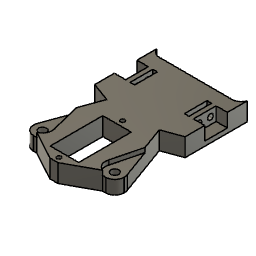
основание (Autodesk Fusion 360 design; units mm, degrees)
Autodesk Fusion 360 part; units mm, degrees
sketch "Sketch1" plane through (0, 0, 0) normal (0, 1, 0) x (1, 0, 0)
  line L0 (-20, 28) -> (20, 28)
  line L1 (20, 28) -> (20, -28)
  line L2 (20, -28) -> (-20, -28)
  line L3 (-20, -28) -> (-20, 28)
  line L4 (-20, 28) -> (20, -28) construction
  line L5 (20, 28) -> (-20, -28) construction
  dimension "d1" = 40
  dimension "d2" = 56
  constraint horizontal L0
  constraint perpendicular L0 L1
  constraint parallel L0 L2
  constraint parallel L1 L3
  constraint coincident L4 origin
  constraint coincident L5 origin
  measures "d1" distance of L1.end L2.end
  measures "d2" distance of L0.end L1.end
extrude "Extrude1" add sketch "Sketch1" along normal blind 8 makes body 1
sketch "Sketch2" plane through (0, 0, -28) normal (0, 0, -1) x (-1, 0, 0)
  line L0 (-20, 0) -> (20, 0)
  line L1 (20, 0) -> (20, 8)
  line L2 (20, 8) -> (-20, 8)
  line L3 (-20, 8) -> (-20, 0)
  line L4 (0, 0) -> (0, 8)
  circle A0 centre (0, 4) radius 2.5
  line L5 (0, 4) -> (-8, 4)
  circle A1 centre (-8, 4) radius 2.5
  line L6 (0, 4) -> (8, 4)
  circle A2 centre (8, 4) radius 2.5
  dimension "d5" = 5
  dimension "d6" = 8
  dimension "d7" = 5
  dimension "d8" = 8
  dimension "d9" = 5
  constraint coincident L4.start origin
  constraint midpoint L2 L4.end
  constraint midpoint L4 A0.centre
  constraint coincident A0.centre L5.start
  constraint perpendicular L4 L5
  constraint coincident L5.end A1.centre
  constraint perpendicular L4 L6
  constraint coincident L6.end A2.centre
  measures "d5" diameter of A0
  measures "d6" distance of A0.centre L5.end
  measures "d7" diameter of A1
  measures "d8" distance of A0.centre L6.end
  measures "d9" diameter of A2
extrude "Extrude2" cut sketch "Sketch2" against normal blind 7 contours L4 A0 L5 | L4 A0 L6 | L4 A0 L5 | L4 A0 L6 | A1 | A2 bodies 1
sketch "Sketch3" plane through (0, 0, -28) normal (0, 0, -1) x (-1, 0, 0)
  circle A0 centre (-8, 4) radius 2.5
  circle A1 centre (0, 4) radius 2.5
  circle A2 centre (8, 4) radius 2.5
  line L0 (-20, 0) -> (20, 0)
  line L1 (20, 0) -> (20, 8)
  line L2 (20, 8) -> (-20, 8)
  line L3 (-20, 8) -> (-20, 0)
  circle A3 centre (-8, 4) radius 3
  circle A4 centre (0, 4) radius 3
  circle A5 centre (8, 4) radius 3
  dimension "d12" = 6
  dimension "d13" = 6
  dimension "d14" = 6
  constraint concentric A0 A3
  constraint concentric A1 A4
  constraint concentric A2 A5
  measures "d12" diameter of A3
  measures "d13" diameter of A4
  measures "d14" diameter of A5
extrude "Extrude3" cut sketch "Sketch3" against normal blind 1 contours A3 | A4 | A5 bodies 1
sketch "Sketch5" plane through (0, 8, 0) normal (0, 1, 0) x (-1, 0, 0)
  line L0 (20, 28) -> (-20, 28)
  line L1 (-20, 28) -> (-20, -28)
  line L2 (-20, -28) -> (20, -28)
  line L3 (20, -28) -> (20, 28)
  line L4 (-20, 28) -> (-20, 18)
  line L5 (-20, 23) -> (-20, 1.5)
  line L6 (-20, 23) -> (-12.6466, 2.7966)
  line L7 (-20, 23) -> (1.5, 23) construction
  line L8 (-20, 28) -> (20, 28)
  line L9 (20, 28) -> (20, 18)
  line L10 (20, 18) -> (-20, 18)
  line L11 (-20, 18) -> (-20, 28)
  line L12 (20, 23) -> (12.6466, 2.7966)
  line L13 (20, 23) -> (-1.5, 23) construction
  line L14 (-12.6466, 2.7966) -> (-11.6205, -0.0225)
  line L15 (12.6466, 2.7966) -> (11.6205, -0.0225)
  line L16 (11.6205, -0.0225) -> (20, -3.0724)
  line L17 (-11.6205, -0.0225) -> (-20, -3.0724)
  dimension "d26" = 10
  dimension "d27" = 21.5
  dimension "d28" = 70
  dimension "d29" = 21.5
  dimension "d30" = 70
  dimension "d31" = 21.5
  dimension "d32" = 3
  dimension "d33" = 3
  constraint coincident L0.end L1.start
  constraint perpendicular L0 L4
  constraint midpoint L4 L5.start
  constraint horizontal L7
  constraint horizontal L8
  constraint vertical L9
  constraint horizontal L10
  constraint vertical L11
  constraint coincident L3 L9.end
  constraint horizontal L13
  constraint midpoint L9 L12.start
  constraint parallel L6 L14
  constraint parallel L12 L15
  constraint coincident L3 L16.end
  constraint perpendicular L15 L16
  constraint coincident L1 L17.end
  constraint perpendicular L14 L17
  measures "d26" distance of L0.end L4.end
  measures "d27" distance of L5.start L5.end
  measures "d28" angle of L6 L7
  measures "d29" distance of L5.start L6.end
  measures "d30" angle of L12 L13
  measures "d31" distance of L12.start L12.end
  measures "d32" distance of L6.end L14.end
  measures "d33" distance of L12.end L15.end
extrude "Extrude5" cut sketch "Sketch5" against normal blind 90 contours L3 L9 L10 L12 | L1 L4 L5 L6 L10 L11 | L3 L10 L12 L15 L16 | L1 L5 L6 L10 L14 L17 bodies 1
sketch "Sketch6" plane through (0, 8, 0) normal (0, 1, 0) x (-1, 0, 0)
  line L0 (-11.6205, -0.0225) -> (-20, -3.0724)
  line L1 (-20, -3.0724) -> (-20, -28)
  line L2 (-20, -28) -> (20, -28)
  line L3 (20, -28) -> (20, -3.0724)
  line L4 (20, -3.0724) -> (11.6205, -0.0225)
  line L5 (11.6205, -0.0225) -> (20, 23)
  line L6 (20, 23) -> (20, 28)
  line L7 (20, 28) -> (-20, 28)
  line L8 (-20, 28) -> (-20, 23)
  line L9 (-20, 23) -> (-11.6205, -0.0225)
  line L10 (-20, 28) -> (-15.9999, 23.9999)
  line L11 (-20, 28) -> (-14.343, 28) construction
  line L12 (20, 28) -> (15.9999, 23.9999)
  line L13 (20, 28) -> (14.343, 28) construction
  circle A0 centre (15.9999, 23.9999) radius 3.15
  circle A1 centre (-15.9999, 23.9999) radius 3.15
  circle A2 centre (15.9999, 23.9999) radius 1.75
  circle A3 centre (-15.9999, 23.9999) radius 1.75
  circle A4 centre (-15.9999, 23.9999) radius 4.0001
  line L14 (-15.9999, 23.9999) -> (-15.9999, 19.9998)
  line L15 (-18.5678, 19.0651) -> (-14.8617, 20.1651)
  circle A5 centre (15.9999, 23.9999) radius 4.0001
  line L16 (15.9999, 23.9999) -> (15.9999, 19.9998)
  line L17 (18.5678, 19.0651) -> (14.8617, 20.1651)
  dimension "d36" = 45
  dimension "d37" = 5.657
  dimension "d38" = 45
  dimension "d39" = 5.657
  dimension "d40" = 6.3
  dimension "d41" = 6.3
  dimension "d42" = 3.5
  dimension "d43" = 3.5
  constraint horizontal L11
  constraint coincident L7.end L8.start
  constraint horizontal L13
  constraint coincident L6.end L7.start
  constraint coincident L12.end A0.centre
  constraint coincident L10.end A1.centre
  constraint concentric A1 A3
  constraint concentric A3 A4
  constraint tangent L7 A4
  constraint coincident A4 L14.end
  constraint vertical L14
  constraint coincident L9 L15.start
  constraint coincident A4 L15.end
  constraint tangent A4 L15
  constraint concentric A0 A5
  constraint tangent L13 A5
  constraint coincident A5 L16.end
  constraint vertical L16
  constraint coincident L5 L17.start
  constraint coincident A5 L17.end
  constraint tangent A5 L17
  measures "d36" angle of L10 L11
  measures "d37" distance of L7.end L10.end
  measures "d38" angle of L12 L13
  measures "d39" distance of L6.end L12.end
  measures "d40" diameter of A0
  measures "d41" diameter of A1
  measures "d42" diameter of A2
  measures "d43" diameter of A3
extrude "Extrude6" cut sketch "Sketch6" against normal blind 6 contours L8 L9 A4 L15 | L10 A1 A4 L14 | L8 L10 A4 | L10 A1 A4 L14 | L7 L10 A4 | L10 A1 A3 L14 | L10 A1 A3 L14 | L10 A3 L14 | L10 A3 L14 | L7 L12 A5 | L12 A0 A5 L16 | L5 L6 A5 L17 | L6 L12 A5 | L12 A0 A5 L16 | L12 A0 A2 L16 | L12 A0 A2 L16 | L12 A2 L16 | L12 A2 L16 bodies 1
extrude "Extrude7" add 2 faces at (-16.9539, 2, 23.7217) (16.9539, 2, 23.7217) along direction (0, -1, 0) blind 4 on bodies 1 bodies 1
extrude "Extrude8" cut 2 faces at (-16.9539, 2, 23.7217) (16.9539, 2, 23.7217) along direction (0, -1, 0) blind 2 on bodies 1 bodies 1
sketch "Sketch7" plane through (0, 0, 0) normal (0, -1, 0) x (1, 0, 0)
  line L0 (18.5678, 19.0651) -> (14.8617, 20.1651)
  arc A0 (15.9999, 28) -> (14.8617, 20.1651) centre (15.9999, 23.9999) ccw
  line L1 (15.9999, 28) -> (-15.9999, 28)
  arc A1 (-14.8617, 20.1651) -> (-15.9999, 28) centre (-15.9999, 23.9999) ccw
  line L2 (-14.8617, 20.1651) -> (-18.5678, 19.0651)
  line L3 (-18.5678, 19.0651) -> (-11.6205, -0.0225)
  line L4 (-11.6205, -0.0225) -> (-20, -3.0724)
  line L5 (-20, -3.0724) -> (-20, -28)
  line L6 (-20, -28) -> (20, -28)
  line L7 (20, -28) -> (20, -3.0724)
  line L8 (20, -3.0724) -> (11.6205, -0.0225)
  line L9 (11.6205, -0.0225) -> (18.5678, 19.0651)
  circle A2 centre (-15.9999, 23.9999) radius 5.5629
  circle A3 centre (15.9999, 23.9999) radius 5.5629
  constraint concentric A1 A2
  constraint coincident L2.end A2
  constraint concentric A0 A3
  constraint coincident L0.start A3
sketch "Sketch10" plane through (0, 8, 0) normal (0, 1, 0) x (-1, 0, 0)
  arc A0 (15.9999, 28) -> (14.8617, 20.1651) centre (15.9999, 23.9999) ccw
  line L0 (15.9999, 28) -> (-15.9999, 28)
  arc A1 (-14.8617, 20.1651) -> (-15.9999, 28) centre (-15.9999, 23.9999) ccw
  line L1 (-14.8617, 20.1651) -> (-18.5678, 19.0651)
  line L2 (-18.5678, 19.0651) -> (-11.6205, -0.0225)
  line L3 (-11.6205, -0.0225) -> (-20, -3.0724)
  line L4 (-20, -3.0724) -> (-20, -28)
  line L5 (-20, -28) -> (20, -28)
  line L6 (20, -28) -> (20, -3.0724)
  line L7 (20, -3.0724) -> (11.6205, -0.0225)
  line L8 (11.6205, -0.0225) -> (18.5678, 19.0651)
  line L9 (18.5678, 19.0651) -> (14.8617, 20.1651)
  line L10 (-20, -28) -> (20, -28)
  line L11 (20, -28) -> (20, -55)
  line L12 (20, -55) -> (-20, -55)
  line L13 (-20, -55) -> (-20, -28)
  constraint horizontal L10
  constraint vertical L11
  constraint horizontal L12
  constraint vertical L13
  constraint coincident L4.end L5.start
extrude "Extrude12" add sketch "Sketch10" against normal blind 7 separate body contours L5 L10 L11 L12 L13 makes body 2
sketch "Sketch11" plane through (0, 8, 0) normal (0, 1, 0) x (-1, 0, 0)
  line L0 (-20, -55) -> (20, -55)
  line L1 (20, -55) -> (20, -28)
  line L2 (20, -28) -> (-20, -28)
  line L3 (-20, -28) -> (-20, -55)
  line L4 (20, -28) -> (15.9999, -32.0001)
  line L5 (20, -28) -> (14.343, -28) construction
  line L6 (-20, -28) -> (-15.9999, -32.0001)
  line L7 (-20, -28) -> (-14.343, -28) construction
  circle A0 centre (15.9999, -32.0001) radius 4.0001
  circle A1 centre (-15.9999, -32.0001) radius 4.0001
  dimension "d63" = 45
  dimension "d64" = 5.657
  dimension "d65" = 5.657
  dimension "d66" = 45
  constraint horizontal L5
  constraint coincident L1.end L2.start
  constraint horizontal L7
  constraint coincident L2.end L3.start
  constraint coincident L4.end A0.centre
  constraint tangent L5 A0
  constraint coincident L6.end A1.centre
  constraint tangent L7 A1
  measures "d63" angle of L4 L5
  measures "d64" distance of L1.end L4.end
  measures "d65" distance of L2.end L6.end
  measures "d66" angle of L6 L7
extrude "Extrude13" cut sketch "Sketch11" against normal blind 25 contours L0 L1 L2 L3 A0 A1 | A1 | A0 bodies 2 makes body 3 at (19.4641, 3.3333, -30.0001)
extrude "Extrude14" add 2 faces at (19.2141, 1, -28.7859) (-19.2141, 1, -28.7859) along direction (0, -1, 0) blind 1 on bodies 2 3 bodies 3 1 2
sketch "Sketch12" plane through (0, 8, 0) normal (0, 1, 0) x (-1, 0, 0)
  arc A0 (-15.9999, -28) -> (-20, -32.0001) centre (-15.9999, -32.0001) ccw
  line L0 (-15.9999, -28) -> (15.9999, -28)
  arc A1 (20, -32.0001) -> (15.9999, -28) centre (15.9999, -32.0001) ccw
  line L1 (20, -32.0001) -> (20, -3.0724)
  line L2 (20, -3.0724) -> (11.6205, -0.0225)
  line L3 (11.6205, -0.0225) -> (18.5678, 19.0651)
  line L4 (18.5678, 19.0651) -> (14.8617, 20.1651)
  arc A2 (15.9999, 28) -> (14.8617, 20.1651) centre (15.9999, 23.9999) ccw
  line L5 (15.9999, 28) -> (-15.9999, 28)
  arc A3 (-14.8617, 20.1651) -> (-15.9999, 28) centre (-15.9999, 23.9999) ccw
  line L6 (-14.8617, 20.1651) -> (-18.5678, 19.0651)
  line L7 (-18.5678, 19.0651) -> (-11.6205, -0.0225)
  line L8 (-11.6205, -0.0225) -> (-20, -3.0724)
  line L9 (-20, -3.0724) -> (-20, -32.0001)
  circle A4 centre (-15.9999, -32.0001) radius 4.25
  circle A5 centre (15.9999, -32.0001) radius 4.25
  dimension "d71" = 8.5
  dimension "d72" = 8.5
  constraint concentric A0 A4
  constraint concentric A1 A5
  measures "d71" diameter of A4
  measures "d72" diameter of A5
extrude "Extrude15" cut sketch "Sketch12" against normal blind 16 contours A0 L0 L9 A4 | L0 A1 L1 A5 picked at (-16.8835, -28.0205) picked at (19.8255, -30.5919) bodies 3
sketch "Sketch13" plane through (0, 8, 0) normal (0, 1, 0) x (-1, 0, 0)
  arc A0 (-14.564, -28) -> (-20, -30.5642) centre (-15.9999, -32.0001) ccw
  line L0 (-14.564, -28) -> (14.564, -28)
  arc A1 (20, -30.5642) -> (14.564, -28) centre (15.9999, -32.0001) ccw
  line L1 (20, -30.5642) -> (20, -3.0724)
  line L2 (20, -3.0724) -> (11.6205, -0.0225)
  line L3 (11.6205, -0.0225) -> (18.5678, 19.0651)
  line L4 (18.5678, 19.0651) -> (14.8617, 20.1651)
  arc A2 (15.9999, 28) -> (14.8617, 20.1651) centre (15.9999, 23.9999) ccw
  line L5 (15.9999, 28) -> (-15.9999, 28)
  arc A3 (-14.8617, 20.1651) -> (-15.9999, 28) centre (-15.9999, 23.9999) ccw
  line L6 (-14.8617, 20.1651) -> (-18.5678, 19.0651)
  line L7 (-18.5678, 19.0651) -> (-11.6205, -0.0225)
  line L8 (-11.6205, -0.0225) -> (-20, -3.0724)
  line L9 (-20, -3.0724) -> (-20, -30.5642)
  line L10 (0, -28) -> (-20, -28)
  line L11 (-15.99, -28) -> (-15.99, -27.7501)
  line L12 (-15.99, -27.7501) -> (-20, -27.7408)
  line L13 (-15.99, -27.7501) -> (20, -27.8339)
  constraint midpoint L0 L10.start
  constraint coincident L9 L10.end
  constraint perpendicular L9 L10
  constraint coincident L10 L11.start
  constraint coincident A0 L11.end
  constraint perpendicular L10 L11
  constraint coincident L9 L12.end
  constraint tangent A0 L12
  constraint coincident L1 L13.end
  constraint tangent A0 L13
extrude "Extrude16" cut sketch "Sketch13" against normal blind 17 contours A0 L0 A1 L10 L13 bodies 3
extrude "Extrude17" cut 3 faces at (-10.8222, 3.851, -27) (-2.8222, 3.851, -27) (5.1871, 3.7268, -27) along direction (0, 0, 1) blind 0.2 on bodies 3 bodies 3
extrude "Extrude18" add 2 faces at (-16.9539, 0, 23.7217) (16.9539, 0, 23.7217) along direction (0, 1, 0) blind 8 on bodies 3 bodies 3
extrude "Extrude19" cut 2 faces at (-16.9539, -2, 23.7217) (16.9539, -2, 23.7217) along direction (0, 1, 0) blind 2 on bodies 3 bodies 3
sketch "Sketch14" plane through (0, 8, 0) normal (0, 1, 0) x (-1, 0, 0)
  line L0 (-15.99, -27.7501) -> (15.2175, -27.8227)
  arc A0 (20, -30.5642) -> (15.2175, -27.8227) centre (15.9999, -32.0001) ccw
  line L1 (20, -30.5642) -> (20, -3.0724)
  line L2 (20, -3.0724) -> (11.6205, -0.0225)
  line L3 (11.6205, -0.0225) -> (20, 23)
  line L4 (20, 23) -> (20, 28)
  line L5 (20, 28) -> (-20, 28)
  line L6 (-20, 28) -> (-20, 23)
  line L7 (-20, 23) -> (-11.6205, -0.0225)
  line L8 (-11.6205, -0.0225) -> (-20, -3.0724)
  line L9 (-20, -3.0724) -> (-20, -30.5642)
  arc A1 (-15.99, -27.7501) -> (-20, -30.5642) centre (-15.9999, -32.0001) ccw
  line L10 (20, 28) -> (15.9999, 23.9999)
  line L11 (20, 28) -> (14.343, 28) construction
  line L12 (-20, 28) -> (-15.9999, 23.9999)
  line L13 (-20, 28) -> (-14.343, 28) construction
  circle A2 centre (15.9999, 23.9999) radius 1.75
  circle A3 centre (-15.9999, 23.9999) radius 1.75
  circle A4 centre (15.9999, 23.9999) radius 4.0001
  circle A5 centre (-15.9999, 23.9999) radius 4.0001
  dimension "d83" = 45
  dimension "d84" = 5.657
  dimension "d85" = 5.657
  dimension "d86" = 45
  dimension "d87" = 3.5
  dimension "d88" = 3.5
  constraint horizontal L11
  constraint coincident L4.end L5.start
  constraint horizontal L13
  constraint coincident L5.end L6.start
  constraint coincident L10.end A2.centre
  constraint coincident L12.end A3.centre
  constraint concentric A2 A4
  constraint tangent L4 A4
  constraint concentric A3 A5
  constraint tangent L6 A5
  measures "d83" angle of L10 L11
  measures "d84" distance of L4.end L10.end
  measures "d85" distance of L5.end L12.end
  measures "d86" angle of L12 L13
  measures "d87" diameter of A2
  measures "d88" diameter of A3
extrude "Extrude20" cut sketch "Sketch14" against normal blind 90 contours L6 L12 A5 | L4 L10 A4 | L5 L12 A5 | L5 L10 A4 | A2 | A3 bodies 3
fillet "Fillet1" radius 5 2 edges at (-20, 4, 23) (20, 4, 23) on bodies 3
sketch "Sketch15" plane through (0, 8, 0) normal (0, 1, 0) x (-1, 0, 0)
  arc A0 (-20, 23.8816) -> (-19.6985, 22.1715) centre (-15, 23.8816) ccw
  line L0 (-19.6985, 22.1715) -> (-11.6205, -0.0225)
  line L1 (-11.6205, -0.0225) -> (-20, -3.0724)
  line L2 (-20, -3.0724) -> (-20, -30.5642)
  arc A1 (-15.99, -27.7501) -> (-20, -30.5642) centre (-15.9999, -32.0001) ccw
  line L3 (-15.99, -27.7501) -> (15.2175, -27.8227)
  arc A2 (20, -30.5642) -> (15.2175, -27.8227) centre (15.9999, -32.0001) ccw
  line L4 (20, -30.5642) -> (20, -3.0724)
  line L5 (20, -3.0724) -> (11.6205, -0.0225)
  line L6 (11.6205, -0.0225) -> (19.6985, 22.1715)
  arc A3 (19.6985, 22.1715) -> (20, 23.8816) centre (15, 23.8816) ccw
  line L7 (20, 23.8816) -> (20, 23.9999)
  arc A4 (20, 23.9999) -> (15.9999, 28) centre (15.9999, 23.9999) ccw
  line L8 (15.9999, 28) -> (-15.9999, 28)
  arc A5 (-15.9999, 28) -> (-20, 23.9999) centre (-15.9999, 23.9999) ccw
  line L9 (-20, 23.9999) -> (-20, 23.8816)
  circle A6 centre (-15.9999, 23.9999) radius 1.75
  circle A7 centre (15.9999, 23.9999) radius 1.75
  circle A8 centre (15.9999, 23.9999) radius 4.25
  circle A9 centre (-15.9999, 23.9999) radius 4.25
  dimension "d94" = 8.5
  dimension "d95" = 8.5
  constraint concentric A4 A8
  constraint concentric A5 A9
  measures "d94" diameter of A8
  measures "d95" diameter of A9
extrude "Extrude21" cut sketch "Sketch15" against normal blind 2 contours A0 L0 L8 A5 L9 A9 | L6 A3 L7 A4 L8 A8 picked at (-15.3915, 27.2353) picked at (15.3915, 27.2353) bodies 3
sketch "Sketch16" plane through (0, 8, 0) normal (0, 1, 0) x (-1, 0, 0)
  arc A0 (14.564, 28) -> (19.4717, 21.5486) centre (15.9999, 23.9999) ccw
  line L0 (14.564, 28) -> (-14.564, 28)
  arc A1 (-19.4717, 21.5486) -> (-14.564, 28) centre (-15.9999, 23.9999) ccw
  line L1 (-19.4717, 21.5486) -> (-11.6205, -0.0225)
  line L2 (-11.6205, -0.0225) -> (-20, -3.0724)
  line L3 (-20, -3.0724) -> (-20, -30.5642)
  arc A2 (-15.99, -27.7501) -> (-20, -30.5642) centre (-15.9999, -32.0001) ccw
  line L4 (-15.99, -27.7501) -> (15.2175, -27.8227)
  arc A3 (20, -30.5642) -> (15.2175, -27.8227) centre (15.9999, -32.0001) ccw
  line L5 (20, -30.5642) -> (20, -3.0724)
  line L6 (20, -3.0724) -> (11.6205, -0.0225)
  line L7 (11.6205, -0.0225) -> (19.4717, 21.5486)
  line L8 (15.9999, 23.9999) -> (11.7499, 23.9999)
  line L9 (15.9999, 23.9999) -> (15.9999, 19.7499)
  line L10 (15.9999, 19.7499) -> (16.5, 19.7499)
  line L11 (16.5, 19.7499) -> (18.8171, 19.7499)
  constraint coincident A0.centre L8.start
  constraint coincident A0 L8.end
  constraint horizontal L8
  constraint coincident A0 L9.end
  constraint perpendicular L8 L9
  constraint tangent A0 L10
  constraint coincident L7 L11.end
  constraint perpendicular L9 L11
extrude "Extrude22" cut sketch "Sketch16" against normal blind 2 contours A0 L7 L10 L11 bodies 3
sketch "Sketch17" plane through (0, 8, 0) normal (0, 1, 0) x (-1, 0, 0)
  line L0 (18.8171, 19.7499) -> (15.9999, 19.7499)
  arc A0 (14.564, 28) -> (15.9999, 19.7499) centre (15.9999, 23.9999) ccw
  line L1 (14.564, 28) -> (-14.564, 28)
  arc A1 (-19.4717, 21.5486) -> (-14.564, 28) centre (-15.9999, 23.9999) ccw
  line L2 (-19.4717, 21.5486) -> (-11.6205, -0.0225)
  line L3 (-11.6205, -0.0225) -> (-20, -3.0724)
  line L4 (-20, -3.0724) -> (-20, -30.5642)
  arc A2 (-15.99, -27.7501) -> (-20, -30.5642) centre (-15.9999, -32.0001) ccw
  line L5 (-15.99, -27.7501) -> (15.2175, -27.8227)
  arc A3 (20, -30.5642) -> (15.2175, -27.8227) centre (15.9999, -32.0001) ccw
  line L6 (20, -30.5642) -> (20, -3.0724)
  line L7 (20, -3.0724) -> (11.6205, -0.0225)
  line L8 (11.6205, -0.0225) -> (18.8171, 19.7499)
  line L9 (-15.9999, 23.9999) -> (-15.9999, 19.7499)
  line L10 (-15.9999, 19.7499) -> (-18.8171, 19.7499)
  constraint coincident A1.centre L9.start
  constraint coincident A1 L9.end
  constraint coincident L2 L10.end
  constraint tangent A1 L10
extrude "Extrude23" cut sketch "Sketch17" against normal blind 2 contours A1 L2 L10 bodies 3
sketch "Sketch18" plane through (0, 8, 0) normal (0, 1, 0) x (-1, 0, 0)
  line L0 (-15.9999, 19.7499) -> (-18.8171, 19.7499)
  line L1 (-18.8171, 19.7499) -> (-11.6205, -0.0225)
  line L2 (-11.6205, -0.0225) -> (-20, -3.0724)
  line L3 (-20, -3.0724) -> (-20, -30.5642)
  arc A0 (-15.99, -27.7501) -> (-20, -30.5642) centre (-15.9999, -32.0001) ccw
  line L4 (-15.99, -27.7501) -> (15.2175, -27.8227)
  arc A1 (20, -30.5642) -> (15.2175, -27.8227) centre (15.9999, -32.0001) ccw
  line L5 (20, -30.5642) -> (20, -3.0724)
  line L6 (20, -3.0724) -> (11.6205, -0.0225)
  line L7 (11.6205, -0.0225) -> (18.8171, 19.7499)
  line L8 (18.8171, 19.7499) -> (15.9999, 19.7499)
  arc A2 (14.564, 28) -> (15.9999, 19.7499) centre (15.9999, 23.9999) ccw
  line L9 (14.564, 28) -> (-14.564, 28)
  arc A3 (-15.9999, 19.7499) -> (-14.564, 28) centre (-15.9999, 23.9999) ccw
  line L10 (-0.3862, -27.7864) -> (20, -27.7864)
  line L11 (20, -27.7864) -> (20.014, -21.7864)
  line L12 (20.014, -21.7864) -> (15.014, -21.7864)
  line L13 (15.014, -21.7864) -> (15.014, -11.7864)
  line L14 (15.014, -11.7864) -> (20.014, -11.7864)
  line L15 (20.014, -11.7864) -> (20.014, -21.7864)
  line L16 (15.014, -21.7864) -> (-20, -21.7864)
  line L17 (-20, -21.7864) -> (-15, -21.7864)
  line L18 (-15, -21.7864) -> (-15, -11.7864)
  line L19 (-15, -11.7864) -> (-20, -11.7864)
  line L20 (-20, -11.7864) -> (-20, -21.7864)
  dimension "d102" = 6
  dimension "d103" = 5
  dimension "d104" = 10
  dimension "d105" = 5
  dimension "d106" = 10
  constraint midpoint L4 L10.start
  constraint coincident L5 L10.end
  constraint perpendicular L5 L10
  constraint perpendicular L4 L11
  constraint horizontal L12
  constraint vertical L13
  constraint horizontal L14
  constraint vertical L15
  constraint coincident L3 L16.end
  constraint perpendicular L3 L16
  constraint horizontal L17
  constraint vertical L18
  constraint horizontal L19
  constraint vertical L20
  measures "d102" distance of L10.end L11.end
  measures "d103" distance of L11.end L12.end
  measures "d104" distance of L11.end L14.end
  measures "d105" distance of L16.end L17.end
  measures "d106" distance of L16.end L19.end
extrude "Extrude24" cut sketch "Sketch18" against normal blind 6 contours L3 L16 L17 L18 L19 L20 | L5 L12 L13 L14 bodies 3
sketch "Sketch19" plane through (-15.014, 0, 0) normal (-1, 0, 0) x (0, 0, 1)
  line L0 (-11.7864, 8) -> (-21.7864, 8)
  line L1 (-21.7864, 8) -> (-21.7864, 2)
  line L2 (-21.7864, 2) -> (-11.7864, 2)
  line L3 (-11.7864, 2) -> (-11.7864, 8)
  line L4 (-21.7864, 8) -> (-21.7864, 2)
  line L5 (-21.7864, 5) -> (-19.2864, 5)
  line L6 (-11.7864, 5) -> (-14.2864, 5)
  circle A0 centre (-19.2864, 5) radius 1.25
  circle A1 centre (-14.2864, 5) radius 1.25
  dimension "d109" = 2.5
  dimension "d110" = 2.5
  dimension "d111" = 2.5
  dimension "d112" = 2.5
  constraint coincident L0.end L1.start
  constraint coincident L1.end L2.start
  constraint midpoint L4 L5.start
  constraint perpendicular L4 L5
  constraint midpoint L3 L6.start
  constraint perpendicular L3 L6
  constraint coincident L5.end A0.centre
  constraint coincident L6.end A1.centre
  measures "d109" distance of L5.start L5.end
  measures "d110" distance of L6.start L6.end
  measures "d111" diameter of A0
  measures "d112" diameter of A1
extrude "Extrude25" cut sketch "Sketch19" against normal blind 4 contours A0 | A1 bodies 3
sketch "Sketch20" plane through (0, 8, 0) normal (0, 1, 0) x (-1, 0, 0)
  line L0 (-20, -11.7864) -> (-15, -11.7864)
  line L1 (-15, -11.7864) -> (-15, -21.7864)
  line L2 (-15, -21.7864) -> (-20, -21.7864)
  line L3 (-20, -21.7864) -> (-20, -30.5642)
  arc A0 (-15.99, -27.7501) -> (-20, -30.5642) centre (-15.9999, -32.0001) ccw
  line L4 (-15.99, -27.7501) -> (15.2175, -27.8227)
  arc A1 (20, -30.5642) -> (15.2175, -27.8227) centre (15.9999, -32.0001) ccw
  line L5 (20, -30.5642) -> (20, -21.7864)
  line L6 (20, -21.7864) -> (15.014, -21.7864)
  line L7 (15.014, -21.7864) -> (15.014, -11.7864)
  line L8 (15.014, -11.7864) -> (20, -11.7864)
  line L9 (20, -11.7864) -> (20, -3.0724)
  line L10 (20, -3.0724) -> (11.6205, -0.0225)
  line L11 (11.6205, -0.0225) -> (18.8171, 19.7499)
  line L12 (18.8171, 19.7499) -> (15.9999, 19.7499)
  arc A2 (14.564, 28) -> (15.9999, 19.7499) centre (15.9999, 23.9999) ccw
  line L13 (14.564, 28) -> (-14.564, 28)
  arc A3 (-15.9999, 19.7499) -> (-14.564, 28) centre (-15.9999, 23.9999) ccw
  line L14 (-15.9999, 19.7499) -> (-18.8171, 19.7499)
  line L15 (-18.8171, 19.7499) -> (-11.6205, -0.0225)
  line L16 (-11.6205, -0.0225) -> (-20, -3.0724)
  line L17 (-20, -3.0724) -> (-20, -11.7864)
  line L18 (20, -21.7864) -> (15.014, -21.7864)
  line L19 (15.014, -21.7864) -> (11.014, -21.7864)
  line L20 (15.014, -21.7864) -> (15.014, -19.2864)
  line L21 (15.014, -19.2864) -> (11.014, -19.2864)
  line L22 (11.014, -19.2864) -> (13.014, -19.2864)
  line L23 (12.014, -19.2864) -> (12.014, -21.7864)
  line L24 (12.014, -21.7864) -> (12.014, -16.7864)
  line L25 (11.014, -21.7864) -> (13.014, -21.7864)
  line L26 (13.014, -21.7864) -> (13.014, -16.7864)
  line L27 (13.014, -16.7864) -> (11.014, -16.7864)
  line L28 (11.014, -16.7864) -> (11.014, -21.7864)
  line L29 (15.014, -11.7864) -> (15.014, -14.2864)
  line L30 (15.014, -14.2864) -> (12.014, -14.2864)
  line L31 (12.014, -14.2864) -> (12.014, -11.7864)
  line L32 (13.014, -11.7864) -> (11.014, -11.7864)
  line L33 (11.014, -11.7864) -> (11.014, -16.7864)
  line L34 (11.014, -16.7864) -> (13.014, -16.7864)
  line L35 (13.014, -16.7864) -> (13.014, -11.7864)
  line L36 (13.014, -11.7864) -> (11.014, -16.7864) construction
  line L37 (11.014, -11.7864) -> (13.014, -16.7864) construction
  point P0 (12.014, -14.2864)
  dimension "d115" = 4
  dimension "d116" = 2.5
  dimension "d117" = 4
  dimension "d118" = 2
  dimension "d119" = 2.5
  dimension "d120" = 5
  dimension "d121" = 2.5
  dimension "d122" = 2.5
  dimension "d123" = 2
  constraint coincident L5.end L6.start
  constraint coincident L6.end L7.start
  constraint perpendicular L5 L19
  constraint perpendicular L6 L20
  constraint perpendicular L20 L21
  constraint parallel L21 L22
  constraint midpoint L22 L23.start
  constraint perpendicular L21 L23
  constraint perpendicular L19 L24
  constraint horizontal L25
  constraint vertical L26
  constraint horizontal L27
  constraint vertical L28
  constraint coincident L7.end L8.start
  constraint perpendicular L8 L29
  constraint perpendicular L29 L30
  constraint perpendicular L30 L31
  constraint horizontal L32
  constraint perpendicular L32 L33
  constraint parallel L32 L34
  constraint parallel L33 L35
  constraint coincident L36 P0
  constraint coincident L37 P0
  constraint coincident P0 L30.end
  measures "d115" distance of L6.end L19.end
  measures "d116" distance of L6.end L20.end
  measures "d117" distance of L20.end L21.end
  measures "d118" distance of L21.end L22.end
  measures "d119" distance of L23.start L23.end
  measures "d120" distance of L23.end L24.end
  measures "d121" distance of L7.end L29.end
  measures "d122" distance of P0 L31.end
  measures "d123" distance of L27.end L26.end
extrude "Extrude26" cut sketch "Sketch20" against normal blind 5 contours L19 L21 L22 L23 L24 L25 L26 | L21 L22 L24 L26 L27 L34 | L19 L21 L22 L23 L24 L25 L28 | L27 L30 L31 L32 L33 L34 L35 | L30 L31 L32 L35 | L21 L22 L24 L27 L28 L34 bodies 3
sketch "Sketch21" plane through (0, 8, 0) normal (0, 1, 0) x (-1, 0, 0)
  line L0 (11.014, -11.7864) -> (13.014, -11.7864)
  line L1 (13.014, -11.7864) -> (13.014, -21.7864)
  line L2 (13.014, -21.7864) -> (11.014, -21.7864)
  line L3 (11.014, -21.7864) -> (11.014, -11.7864)
  line L4 (-20, -11.7864) -> (-15, -11.7864)
  line L5 (-15, -11.7864) -> (-15, -21.7864)
  line L6 (-15, -21.7864) -> (-20, -21.7864)
  line L7 (-20, -21.7864) -> (-20, -30.5642)
  arc A0 (-15.99, -27.7501) -> (-20, -30.5642) centre (-15.9999, -32.0001) ccw
  line L8 (-15.99, -27.7501) -> (15.2175, -27.8227)
  arc A1 (20, -30.5642) -> (15.2175, -27.8227) centre (15.9999, -32.0001) ccw
  line L9 (20, -30.5642) -> (20, -21.7864)
  line L10 (20, -21.7864) -> (15.014, -21.7864)
  line L11 (15.014, -21.7864) -> (15.014, -11.7864)
  line L12 (15.014, -11.7864) -> (20, -11.7864)
  line L13 (20, -11.7864) -> (20, -3.0724)
  line L14 (20, -3.0724) -> (11.6205, -0.0225)
  line L15 (11.6205, -0.0225) -> (18.8171, 19.7499)
  line L16 (18.8171, 19.7499) -> (15.9999, 19.7499)
  arc A2 (14.564, 28) -> (15.9999, 19.7499) centre (15.9999, 23.9999) ccw
  line L17 (14.564, 28) -> (-14.564, 28)
  arc A3 (-15.9999, 19.7499) -> (-14.564, 28) centre (-15.9999, 23.9999) ccw
  line L18 (-15.9999, 19.7499) -> (-18.8171, 19.7499)
  line L19 (-18.8171, 19.7499) -> (-11.6205, -0.0225)
  line L20 (-11.6205, -0.0225) -> (-20, -3.0724)
  line L21 (-20, -3.0724) -> (-20, -11.7864)
  line L22 (-15, -16.7864) -> (-13, -16.7864)
  line L23 (-13, -16.7864) -> (-13, -11.7864)
  line L24 (-13, -11.7864) -> (-11, -11.7864)
  line L25 (-11, -11.7864) -> (-11, -21.7864)
  line L26 (-11, -21.7864) -> (-13, -21.7864)
  line L27 (-13, -21.7864) -> (-13, -11.7864)
  dimension "d126" = 2
  dimension "d127" = 2
  dimension "d128" = 10
  constraint midpoint L5 L22.start
  constraint perpendicular L5 L22
  constraint perpendicular L22 L23
  constraint horizontal L24
  constraint vertical L25
  constraint horizontal L26
  constraint vertical L27
  measures "d126" distance of L22.start L22.end
  measures "d127" distance of L23.end L24.end
  measures "d128" distance of L23.end L26.end
extrude "Extrude27" cut sketch "Sketch21" against normal blind 5 contours L23 L24 L25 L26 L27 bodies 3
sketch "Sketch22" plane through (15, 0, 0) normal (1, 0, 0) x (0, 0, -1)
  line L0 (21.7864, 8) -> (11.7864, 8)
  line L1 (11.7864, 8) -> (11.7864, 2)
  line L2 (11.7864, 2) -> (21.7864, 2)
  line L3 (21.7864, 2) -> (21.7864, 8)
  line L4 (11.7864, 5) -> (14.2864, 5)
  circle A0 centre (14.2864, 5) radius 1.25
  line L5 (21.7864, 5) -> (19.2864, 5)
  circle A1 centre (19.2864, 5) radius 1.25
  dimension "d131" = 2.5
  dimension "d132" = 2.5
  dimension "d133" = 2.5
  dimension "d134" = 2.5
  constraint midpoint L1 L4.start
  constraint perpendicular L1 L4
  constraint coincident L4.end A0.centre
  constraint midpoint L3 L5.start
  constraint perpendicular L3 L5
  constraint coincident L5.end A1.centre
  measures "d131" distance of L4.start L4.end
  measures "d132" diameter of A0
  measures "d133" distance of L5.start L5.end
  measures "d134" diameter of A1
extrude "Extrude28" cut sketch "Sketch22" against normal blind 4 contours A0 | A1 bodies 3
sketch "Sketch23" plane through (0, 8, 0) normal (0, 1, 0) x (-1, 0, 0)
  line L0 (-11, -11.7864) -> (-11, -21.7864)
  line L1 (-11, -21.7864) -> (-13, -21.7864)
  line L2 (-13, -21.7864) -> (-13, -11.7864)
  line L3 (-13, -11.7864) -> (-11, -11.7864)
  line L4 (11.014, -11.7864) -> (13.014, -11.7864)
  line L5 (13.014, -11.7864) -> (13.014, -21.7864)
  line L6 (13.014, -21.7864) -> (11.014, -21.7864)
  line L7 (11.014, -21.7864) -> (11.014, -11.7864)
  line L8 (-20, -11.7864) -> (-15, -11.7864)
  line L9 (-15, -11.7864) -> (-15, -21.7864)
  line L10 (-15, -21.7864) -> (-20, -21.7864)
  line L11 (-20, -21.7864) -> (-20, -30.5642)
  arc A0 (-15.99, -27.7501) -> (-20, -30.5642) centre (-15.9999, -32.0001) ccw
  line L12 (-15.99, -27.7501) -> (15.2175, -27.8227)
  arc A1 (20, -30.5642) -> (15.2175, -27.8227) centre (15.9999, -32.0001) ccw
  line L13 (20, -30.5642) -> (20, -21.7864)
  line L14 (20, -21.7864) -> (15.014, -21.7864)
  line L15 (15.014, -21.7864) -> (15.014, -11.7864)
  line L16 (15.014, -11.7864) -> (20, -11.7864)
  line L17 (20, -11.7864) -> (20, -3.0724)
  line L18 (20, -3.0724) -> (11.6205, -0.0225)
  line L19 (11.6205, -0.0225) -> (18.8171, 19.7499)
  line L20 (18.8171, 19.7499) -> (15.9999, 19.7499)
  arc A2 (14.564, 28) -> (15.9999, 19.7499) centre (15.9999, 23.9999) ccw
  line L21 (14.564, 28) -> (-14.564, 28)
  arc A3 (-15.9999, 19.7499) -> (-14.564, 28) centre (-15.9999, 23.9999) ccw
  line L22 (-15.9999, 19.7499) -> (-18.8171, 19.7499)
  line L23 (-18.8171, 19.7499) -> (-11.6205, -0.0225)
  line L24 (-11.6205, -0.0225) -> (-20, -3.0724)
  line L25 (-20, -3.0724) -> (-20, -11.7864)
  line L26 (-11.8128, 23.2712) -> (-15.2188, 9.8637)
  line L27 (11.8128, 23.2712) -> (15.2188, 9.8637)
  constraint midpoint A3 L26.start
  constraint midpoint L23 L26.end
  constraint midpoint A2 L27.start
  constraint midpoint L19 L27.end
extrude "Extrude29" cut sketch "Sketch23" against normal blind 2 contours A3 L22 L23 L26 | L19 L20 A2 L27 bodies 3
sketch "Sketch24" plane through (0, 0, 0) normal (0, -1, 0) x (1, 0, 0)
  arc A0 (19.6985, 22.1715) -> (20, 23.8816) centre (15, 23.8816) ccw
  line L0 (20, 23.8816) -> (20, 23.9999)
  arc A1 (20, 23.9999) -> (15.9999, 28) centre (15.9999, 23.9999) ccw
  line L1 (15.9999, 28) -> (-15.9999, 28)
  arc A2 (-15.9999, 28) -> (-20, 23.9999) centre (-15.9999, 23.9999) ccw
  line L2 (-20, 23.9999) -> (-20, 23.8816)
  arc A3 (-20, 23.8816) -> (-19.6985, 22.1715) centre (-15, 23.8816) ccw
  line L3 (-19.6985, 22.1715) -> (-11.6205, -0.0225)
  line L4 (-11.6205, -0.0225) -> (-20, -3.0724)
  line L5 (-20, -3.0724) -> (-20, -30.5642)
  arc A4 (-15.2175, -27.8227) -> (-20, -30.5642) centre (-15.9999, -32.0001) ccw
  line L6 (-15.2175, -27.8227) -> (15.99, -27.7501)
  arc A5 (20, -30.5642) -> (15.99, -27.7501) centre (15.9999, -32.0001) ccw
  line L7 (20, -30.5642) -> (20, -3.0724)
  line L8 (20, -3.0724) -> (11.6205, -0.0225)
  line L9 (11.6205, -0.0225) -> (19.6985, 22.1715)
  circle A6 centre (-15.9999, 23.9999) radius 1.75
  circle A7 centre (15.9999, 23.9999) radius 1.75
  line L10 (-18.9999, 22.2678) -> (-15.9999, 20.5358)
  line L11 (-15.9999, 20.5358) -> (-12.9999, 22.2678)
  line L12 (-12.9999, 22.2678) -> (-12.9999, 25.7319)
  line L13 (-12.9999, 25.7319) -> (-15.9999, 27.464)
  line L14 (-15.9999, 27.464) -> (-18.9999, 25.7319)
  line L15 (-18.9999, 25.7319) -> (-18.9999, 22.2678)
  line L16 (12.9999, 22.2678) -> (15.9999, 20.5358)
  line L17 (15.9999, 20.5358) -> (18.9999, 22.2678)
  line L18 (18.9999, 22.2678) -> (18.9999, 25.7319)
  line L19 (18.9999, 25.7319) -> (15.9999, 27.464)
  line L20 (15.9999, 27.464) -> (12.9999, 25.7319)
  line L21 (12.9999, 25.7319) -> (12.9999, 22.2678)
  point P0 (-15.9999, 23.9999)
  point P1 (15.9999, 23.9999)
  dimension "d139" = 3
  dimension "d140" = 3
  constraint coincident P0 A2.centre
  constraint coincident P1 A1.centre
  measures "d139" distance of P0 L15
  measures "d140" distance of P1 L21
extrude "Extrude30" cut sketch "Sketch24" against normal blind 2 contours L10 L11 L12 L13 L14 L15 | L16 L17 L18 L19 L20 L21 bodies 3
sketch "Sketch25" plane through (0, 8, 0) normal (0, 1, 0) x (-1, 0, 0)
  line L0 (-11.9727, 22.6419) -> (-15.2188, 9.8637)
  line L1 (-15.2188, 9.8637) -> (-11.6205, -0.0225)
  line L2 (-11.6205, -0.0225) -> (-20, -3.0724)
  line L3 (-20, -3.0724) -> (-20, -11.7864)
  line L4 (-20, -11.7864) -> (-15, -11.7864)
  line L5 (-15, -11.7864) -> (-15, -21.7864)
  line L6 (-15, -21.7864) -> (-20, -21.7864)
  line L7 (-20, -21.7864) -> (-20, -30.5642)
  arc A0 (-15.99, -27.7501) -> (-20, -30.5642) centre (-15.9999, -32.0001) ccw
  line L8 (-15.99, -27.7501) -> (15.2175, -27.8227)
  arc A1 (20, -30.5642) -> (15.2175, -27.8227) centre (15.9999, -32.0001) ccw
  line L9 (20, -30.5642) -> (20, -21.7864)
  line L10 (20, -21.7864) -> (15.014, -21.7864)
  line L11 (15.014, -21.7864) -> (15.014, -11.7864)
  line L12 (15.014, -11.7864) -> (20, -11.7864)
  line L13 (20, -11.7864) -> (20, -3.0724)
  line L14 (20, -3.0724) -> (11.6205, -0.0225)
  line L15 (11.6205, -0.0225) -> (15.2188, 9.8637)
  line L16 (15.2188, 9.8637) -> (11.9727, 22.6419)
  arc A2 (14.564, 28) -> (11.9727, 22.6419) centre (15.9999, 23.9999) ccw
  line L17 (14.564, 28) -> (-14.564, 28)
  arc A3 (-11.9727, 22.6419) -> (-14.564, 28) centre (-15.9999, 23.9999) ccw
  line L18 (-11, -11.7864) -> (-11, -21.7864)
  line L19 (-11, -21.7864) -> (-13, -21.7864)
  line L20 (-13, -21.7864) -> (-13, -11.7864)
  line L21 (-13, -11.7864) -> (-11, -11.7864)
  line L22 (11.014, -11.7864) -> (13.014, -11.7864)
  line L23 (13.014, -11.7864) -> (13.014, -21.7864)
  line L24 (13.014, -21.7864) -> (11.014, -21.7864)
  line L25 (11.014, -21.7864) -> (11.014, -11.7864)
  line L26 (15.9999, 23.9999) -> (-15.9999, 23.9999)
  line L27 (0, 23.9999) -> (0, 33.3999)
  line L28 (0, 33.3999) -> (0, 35.3999)
  line L29 (0, 35.3999) -> (0, 28)
  circle A4 centre (0, 31.6999) radius 3.6999
  line L30 (14.564, 28) -> (1.7659, 34.9513)
  line L31 (-14.564, 28) -> (-1.7659, 34.9513)
  line L32 (1.7659, 34.9513) -> (-1.7659, 34.9513)
  dimension "d143" = 9.4
  dimension "d144" = 2
  constraint coincident A2.centre L26.start
  constraint coincident A3.centre L26.end
  constraint midpoint L26 L27.start
  constraint perpendicular L17 L27
  constraint vertical L28
  constraint midpoint L17 L29.end
  constraint midpoint L29 A4.centre
  constraint coincident L29.end A4
  constraint coincident A2.start L17.start
  constraint coincident A4 L30.end
  constraint tangent A4 L30
  constraint coincident L17.end A3.end
  constraint coincident A4 L31.end
  constraint tangent A4 L31
  measures "d143" distance of L27.start L27.end
  measures "d144" distance of L27.end L28.end
extrude "Extrude31" add sketch "Sketch25" against normal blind 8 contours L17 A4 L31 | L17 A4 L30 | L27 L28 L29 A4 L32 | L27 L28 L29 A4 L32 bodies 3
sketch "Sketch26" plane through (0, 8, 0) normal (0, 1, 0) x (-1, 0, 0)
  line L0 (-11.9727, 22.6419) -> (-15.2188, 9.8637)
  line L1 (-15.2188, 9.8637) -> (-11.6205, -0.0225)
  line L2 (-11.6205, -0.0225) -> (-20, -3.0724)
  line L3 (-20, -3.0724) -> (-20, -11.7864)
  line L4 (-20, -11.7864) -> (-15, -11.7864)
  line L5 (-15, -11.7864) -> (-15, -21.7864)
  line L6 (-15, -21.7864) -> (-20, -21.7864)
  line L7 (-20, -21.7864) -> (-20, -30.5642)
  arc A0 (-15.99, -27.7501) -> (-20, -30.5642) centre (-15.9999, -32.0001) ccw
  line L8 (-15.99, -27.7501) -> (15.2175, -27.8227)
  arc A1 (20, -30.5642) -> (15.2175, -27.8227) centre (15.9999, -32.0001) ccw
  line L9 (20, -30.5642) -> (20, -21.7864)
  line L10 (20, -21.7864) -> (15.014, -21.7864)
  line L11 (15.014, -21.7864) -> (15.014, -11.7864)
  line L12 (15.014, -11.7864) -> (20, -11.7864)
  line L13 (20, -11.7864) -> (20, -3.0724)
  line L14 (20, -3.0724) -> (11.6205, -0.0225)
  line L15 (11.6205, -0.0225) -> (15.2188, 9.8637)
  line L16 (15.2188, 9.8637) -> (11.9727, 22.6419)
  arc A2 (14.564, 28) -> (11.9727, 22.6419) centre (15.9999, 23.9999) ccw
  line L17 (14.564, 28) -> (1.7659, 34.9513)
  line L18 (1.7659, 34.9513) -> (-1.7659, 34.9513)
  line L19 (-1.7659, 34.9513) -> (-14.564, 28)
  arc A3 (-11.9727, 22.6419) -> (-14.564, 28) centre (-15.9999, 23.9999) ccw
  line L20 (-11, -11.7864) -> (-11, -21.7864)
  line L21 (-11, -21.7864) -> (-13, -21.7864)
  line L22 (-13, -21.7864) -> (-13, -11.7864)
  line L23 (-13, -11.7864) -> (-11, -11.7864)
  line L24 (11.014, -11.7864) -> (13.014, -11.7864)
  line L25 (13.014, -11.7864) -> (13.014, -21.7864)
  line L26 (13.014, -21.7864) -> (11.014, -21.7864)
  line L27 (11.014, -21.7864) -> (11.014, -11.7864)
  line L28 (15.9999, 23.9999) -> (-15.9999, 23.9999)
  circle A4 centre (0, 23.9999) radius 6.3
  line L29 (0, 23.9999) -> (0, 30.2999)
  line L30 (0, 30.2999) -> (0, 7.0499)
  line L31 (6.3, 7.0499) -> (-6.3, 7.0499)
  line L32 (-6.3, 7.0499) -> (-6.3, 30.2999)
  line L33 (-6.3, 30.2999) -> (6.3, 30.2999)
  line L34 (6.3, 30.2999) -> (6.3, 7.0499)
  line L35 (6.3, 7.0499) -> (-6.3, 30.2999) construction
  line L36 (-6.3, 7.0499) -> (6.3, 30.2999) construction
  line L37 (0, 7.0499) -> (0, 5.5499)
  line L38 (0, 30.2999) -> (0, 31.7999)
  line L39 (0, 31.7999) -> (0, 33.6999)
  circle A5 centre (0, 32.7499) radius 0.95
  line L40 (0, 5.5499) -> (0, 3.6499)
  circle A6 centre (0, 4.5999) radius 0.95
  point P0 (0, 18.6749)
  dimension "d147" = 12.6
  dimension "d148" = 23.25
  dimension "d149" = 12.6
  dimension "d150" = 1.5
  dimension "d151" = 1.5
  dimension "d152" = 1.9
  dimension "d153" = 1.9
  constraint coincident A2.centre L28.start
  constraint coincident A3.centre L28.end
  constraint midpoint L28 A4.centre
  constraint coincident A4.centre L29.start
  constraint coincident A4 L29.end
  constraint perpendicular L28 L29
  constraint perpendicular L28 L30
  constraint horizontal L31
  constraint perpendicular L31 L32
  constraint parallel L31 L33
  constraint parallel L32 L34
  constraint coincident L35 P0
  constraint coincident L36 P0
  constraint midpoint L30 P0
  constraint perpendicular L31 L37
  constraint perpendicular L33 L38
  constraint parallel L38 L39
  constraint midpoint L39 A5.centre
  constraint coincident L39.end A5
  constraint parallel L37 L40
  constraint midpoint L40 A6.centre
  constraint coincident L40.end A6
  measures "d147" diameter of A4
  measures "d148" distance of L29.end L30.end
  measures "d149" distance of L32.end L33.end
  measures "d150" distance of L30.end L37.end
  measures "d151" distance of L29.end L38.end
  measures "d152" distance of L38.end L39.end
  measures "d153" distance of L37.end L40.end
extrude "Extrude32" cut sketch "Sketch26" against normal blind 90 contours L28 A4 L29 L30 | A4 L32 L33 | L28 A4 L30 | A4 L30 L31 L32 | L28 A4 L29 L30 | L28 A4 L30 | A4 L33 L34 | A4 L30 L31 L34 | L39 A5 | L39 A5 | L40 A6 | L40 A6 bodies 3
equation "d27 = ( 43 / 2 ) * 1 mm"
equation "d143 = 6 mm + 1.5 mm + 1.9 mm"
